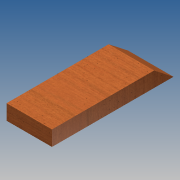
# Autodesk Inventor part: 2p2psh3
Saved by Autodesk Inventor 2014 SP1 (Build 180222100, 222)
## iProperties
Company: HERA Project
Created: 2013-09-03
Part Number: 2p2psh3
Material: Wood (Cherry)
Document SubType Name: Modeling
Designer: David DeBoer
Mass: 474.148 g
Surface Area: 800.643 cm^2
Volume: 948.296 cm^3
Density: 0.5 g/cm^3
Description: Pole stand support horizontal 3
Appearance: Cherry - Natural Low Gloss
Author: David DeBoer
Autodesk Inventor part; units mm, degrees
ref_plane "YZ Plane" through (0, 0, 0) normal (1, 0, 0) x (0, 1, 0)
ref_plane "XZ Plane" through (0, 0, 0) normal (0, 1, 0) x (-1, 0, 0)
ref_plane "XY Plane" through (0, 0, 0) normal (0, 0, 1) x (1, 0, 0)
sketch "Sketch1" plane through (0, 0, 0) normal (1, 0, 0) x (0, 1, 0)
  line L0 (0, 0) -> (38, 0)
  line L1 (38, 0) -> (38, -256.1622)
  line L2 (38.1, -304.8) -> (0, -304.8) construction
  line L3 (0, -304.8) -> (0, 0)
  line L4 (0, -304.8) -> (38, -256.1622)
  dimension "d0" = 38
  dimension "d1" = 304.8
  dimension "d2" = 38
  constraints: 10 end point, 2 parallel, 1 horizontal, 1 perpendicular
  measures "d0" distance of L0.start L0.end
  measures "d1" distance of L2.end L0.start
  measures "d2" angle of L4 L3
extrude "Extrusion1" add sketch "Sketch1" along normal blind 114
body "Solid1"
